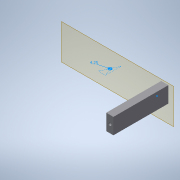
# Autodesk Inventor part: coupler
Saved by Autodesk Inventor 2020 (Build 240168000, 168)
## iProperties
Created: 2020-05-14
Part Number: coupler
Material: Ogólny
Document SubType Name: Modeling
Designer: blep
Density: 1 g/cm^3
Appearance: Domyślna
Author: blep
Autodesk Inventor part; units mm, degrees
ref_plane "YZ Plane" through (0, 0, 0) normal (1, 0, 0) x (0, 1, 0)
ref_plane "XZ Plane" through (0, 0, 0) normal (0, 1, 0) x (-1, 0, 0)
ref_plane "XY Plane" through (0, 0, 0) normal (0, 0, 1) x (1, 0, 0)
ref_plane "Płaszczyzna konstrukcyjna1" through (0, 0, 0) normal (0, 0, 1) x (1, 0, 0)
sketch "Szkic1" plane through (0, 0, 0) normal (0, 0, 1) x (1, 0, 0)
  line L0 (60.3592, 11) -> (60.3592, -11) projected
  line L1 (70.3592, 11) -> (70.3592, -11) projected
  line L2 (70.3592, -11) -> (60.3592, -11)
  line L3 (60.3592, -11) -> (60.3592, 11)
  line L4 (60.3592, 11) -> (70.3592, 11)
  line L5 (70.3592, 11) -> (70.3592, -11)
  point P0 (0, 0)
  constraints: 8 end point, 2 parallel, 1 horizontal, 1 perpendicular
extrude "Wyciągnięcie proste1" add sketch "Szkic1" along normal blind 76
sketch "Szkic2" plane through (0, 0, 0) normal (0, 0, -1) x (-1, 0, 0)
  circle A0 centre (-65.3592, 0) radius 2.125
  line L0 (-70.3592, 11) -> (-60.3592, 11) construction
  line L1 (-65.3592, 0) -> (-70.3592, 11) construction
  line L2 (-60.3592, 11) -> (-65.3592, 0) construction
  line L3 (-60.3592, 11) -> (-60.3592, -11) construction
  line L4 (-65.3592, 0) -> (-60.3592, -11) construction
  point P0 (0, 0)
  dimension "d13" = 4.25
  constraints: 6 end point, 2 equal length, 1 centre point
  measures "d13" diameter of A0
extrude "Wyciągnięcie proste3" cut sketch "Szkic2" against normal through all
sketch "Szkic3" plane through (70.3592, -11, 0) normal (1, 0, 0) x (0, 0, -1)
  line L0 (-66, 15) -> (-62.5, 15)
  line L1 (-62.5, 15) -> (-62.5, 7)
  line L2 (-62.5, 7) -> (-66, 7)
  line L3 (-66, 7) -> (-66, 15)
  line L4 (-13.5, 15) -> (-10, 15)
  line L5 (-10, 15) -> (-10, 7)
  line L6 (-10, 7) -> (-13.5, 7)
  line L7 (-13.5, 7) -> (-13.5, 15)
  line L8 (0, 22) -> (-76, 22) projected
  line L9 (0, 0) -> (-76, 0) projected
  line L10 (-76, 0) -> (-76, 22) projected
  line L11 (0, 0) -> (0, 22) projected
  line L12 (-66, 22) -> (-66, 15) construction
  line L13 (-66, 0) -> (-66, 7) construction
  point P0 (0, 11)
  dimension "d2" = 10
  dimension "d3" = 10
  dimension "d4" = 3.5
  dimension "d6" = 8
  dimension "d7" = 3.5
  constraints: 20 end point, 4 parallel, 4 point on line, 2 horizontal, 2 perpendicular, 2 vertical, 1 collinear
  measures "d2" distance between parallel lines of L3 L10
  measures "d3" distance between parallel lines of L5 L11
  measures "d4" distance between parallel lines of L1 L3
  measures "d6" distance between parallel lines of L2 L0
  measures "d7" distance of L5.end L6.end
equation "\"d3\" = d2"
equation "\"d7\" = d4"
